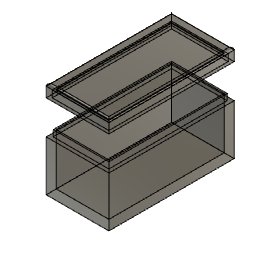
Box Attempt 2 v1 (Autodesk Fusion 360 design; units mm, degrees)
Autodesk Fusion 360 part; units mm, degrees
sketch "Sketch1" plane through (0, 0, 0) normal (0, 1, 0) x (1, 0, 0)
  line L0 (0, 0) -> (50, 0)
  line L1 (50, 0) -> (50, -50)
  line L2 (50, -50) -> (0, -50)
  line L3 (0, -50) -> (0, 0)
  constraint horizontal L0
  constraint vertical L1
  constraint horizontal L2
  constraint vertical L3
  constraint coincident L0.start L3.end
extrude "Extrude1" add sketch "Sketch1" along normal blind 100 makes body 1
shell "Shell1" thickness 4 removed faces 0 bodies 1
ref_plane "WorkPlane1" through (0, 0, 40) normal (0, 0, 1) x (1, 0, 0)
move_body "Move1" bodies 1 to x (1, 0, 0) y (0, 1, 0) z (0, 0, 1) at (0, 20, 0)
split "Split1" by plane through (0, 0, 40) normal (0, 0, 1) bodies 1 makes body 2 at (33.3333, 53.3333, 50)
sketch "Sketch2" plane through (0, 0, 40) normal (0, 0, 1) x (-1, 0, 0)
  line L0 (-50, -20) -> (-50, -120)
  line L1 (-50, -120) -> (0, -120)
  line L2 (0, -120) -> (0, -20)
  line L3 (0, -20) -> (-50, -20)
  line L4 (-46, -116) -> (-46, -24)
  line L5 (-46, -24) -> (-4, -24)
  line L6 (-4, -24) -> (-4, -116)
  line L7 (-4, -116) -> (-46, -116)
  line L8 (-47.2, -117.2) -> (-47.2, -22.8)
  line L9 (-47.2, -22.8) -> (-2.8, -22.8)
  line L10 (-2.8, -22.8) -> (-2.8, -117.2)
  line L11 (-2.8, -117.2) -> (-47.2, -117.2)
  dimension "d6" = -1.2
extrude "Extrude2" add sketch "Sketch2" along normal blind 5 contours L8 L9 L10 L11 bodies 1
combine "Combine1" operation cut target body 2 tool bodies 1 keep tools
move_face "OffsetFaces1" offset -0.4 5 faces at (47.2, 85.7333, 41.6667) (3.2, 54.6667, 45) (17.6, 117.2, 41.6667) (32.4, 22.8, 41.6667) (2.8, 54.2667, 41.6667) on bodies 2
copy_body "Body->Comp1" bodies 1 removing the originals makes body 3 in component "Box"
copy_body "Body->Comp2" bodies 2 removing the originals makes body 4 in component "Lid"
move_body "Move1'" bodies 4 to x (1, 0, 0) y (0, 1, 0) z (0, 0, 1) at (0, 0, 16) in component "Lid"
move_body "Move2" bodies 4 to x (1, 0, 0) y (0, 1, 0) z (0, 0, 1) at (0, 0, -2) in component "Lid"
fillet "Fillet1" radius 2 4 edges at (25, 120, 64) (0, 70, 64) (25, 20, 64) (50, 70, 64) on bodies 4 in component "Lid"
component "Box" placed x (1, 0, 0) y (0, 1, 0) z (0, 0, 1) at (0, 0, 0)
component "Lid" placed x (1, 0, 0) y (0, 1, 0) z (0, 0, 1) at (0, 0, 0)
